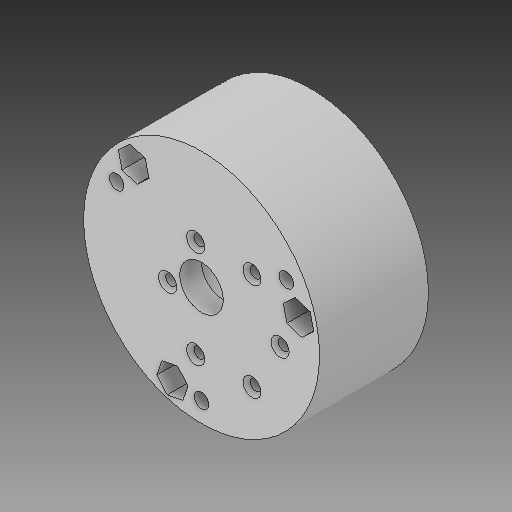
# Autodesk Inventor part: наболдашник
Saved by Autodesk Inventor 2019 (Build 230136000, 136)
## iProperties
Created: 2018-01-15
Part Number: наболдашник
Material: Типовые
Document SubType Name: Modeling
Designer: olege
Density: 1 g/cm^3
Appearance: По умолчанию
Mass: 53.9345 g
Surface Area: 284.424 cm^2
Volume: 53.9345 cm^3
Author: olege
Autodesk Inventor part; units mm, degrees
ref_plane "YZ Plane" through (0, 0, 0) normal (1, 0, 0) x (0, 1, 0)
ref_plane "XZ Plane" through (0, 0, 0) normal (0, 1, 0) x (-1, 0, 0)
ref_plane "XY Plane" through (0, 0, 0) normal (0, 0, 1) x (1, 0, 0)
sketch "Эскиз1" plane through (0, 0, 0) normal (0, 0, 1) x (1, 0, 0)
  circle A0 centre (0, 0) radius 18.65
  circle A1 centre (0, 0) radius 20.5
  dimension "d0" = 37.3
  dimension "d1" = 41
  constraints: 2 centre point, 2 coincident
  measures "d0" diameter of A0
  measures "d1" diameter of A1
extrude "Выдавливание1" add sketch "Эскиз1" against normal blind 24
sketch "Эскиз2" plane through (0, 0, 0) normal (0, 0, 1) x (1, 0, 0)
  circle A0 centre (0, 0) radius 20.5
  dimension "d4" = 41
  constraints: 1 centre point, 1 coincident
  measures "d4" diameter of A0
extrude "Выдавливание2" add sketch "Эскиз2" along normal blind 2
sketch "Эскиз3" plane through (0, 0, 2) normal (0, 0, 1) x (1, 0, 0)
  circle A0 centre (15.5, 0) radius 1.5
  point P0 (0, 0)
  dimension "d9" = 3
  dimension "d10" = 15.5
  constraints: 1 centre point, 1 horizontal alignment
  measures "d9" diameter of A0
  measures "d10" distance of point (0, 0) A0.centre
extrude "Выдавливание3" cut sketch "Эскиз3" against normal blind 2
pattern_circular "Круговой массив1" count 6 over 360 about axis through (0, 0, 0) along (0, 0, -1) of "Выдавливание3"
sketch "Эскиз4" plane through (0, 0, 2) normal (0, 0, 1) x (1, 0, 0)
  circle A0 centre (-6.1423, 3.3574) radius 6
  circle A1 centre (-7.75, 13.4234) radius 1.5 projected
  point P0 (0, 0)
  dimension "d17" = 12
  dimension "d19" = 7
  dimension "d20" = 10.066
  constraints: 1 centre point
  measures "d17" diameter of A0
  measures "d19" distance of point (0, 0) A0.centre
  measures "d20" vertical distance of A0.centre A1.centre
extrude "Выдавливание4" cut sketch "Эскиз4" against normal blind 2 contours A0
sketch "Эскиз5" plane through (0, 0, 2) normal (0, 0, 1) x (1, 0, 0)
  circle A0 centre (-6.1423, 3.3574) radius 6 construction
  circle A1 centre (-6.1423, 3.3574) radius 32.5
  circle A2 centre (0, 0) radius 20.5 projected
  dimension "d48" = 65
  constraints: 1 centre point, 1 coincident
  measures "d48" diameter of A1
extrude "Выдавливание5" add sketch "Эскиз5" against normal blind 2
sketch "Эскиз6" plane through (-6.1423, 3.3574, 0) normal (0, 0, -1) x (-1, 0, 0)
  circle A0 centre (0, 0) radius 32.5
  circle A1 centre (0, 0) radius 25.5
  point P0 (-6.1423, -3.3574)
  dimension "d25" = 51
  dimension "d26" = 65
  constraints: 2 centre point, 1 coincident
  measures "d25" diameter of A1
  measures "d26" diameter of A0
extrude "Выдавливание6" add sketch "Эскиз6" along normal blind 24
sketch "Эскиз8" plane through (0, 0, -24) normal (0, 0, -1) x (-1, 0, 0)
  circle A0 centre (0, 0) radius 18.65
  circle A1 centre (6.1423, 3.3574) radius 6 projected
  circle A2 centre (6.1423, 3.3574) radius 32.5
  circle A3 centre (6.1423, 3.3574) radius 35
  dimension "d33" = 65
  dimension "d34" = 70
  dimension "d209" = 37.3
  constraints: 3 centre point, 3 coincident
  measures "d33" diameter of A2
  measures "d34" diameter of A3
  measures "d209" diameter of A0
extrude "Выдавливание7" cut sketch "Эскиз8" against normal blind 25 contours A0 | A1 | A3
sketch "Эскиз10" plane through (0, 0, 1) normal (0, 0, -1) x (-1, 0, 0)
  circle A0 centre (6.1423, 3.3574) radius 6 projected
  circle A1 centre (-7.75, 13.4234) radius 1.5 projected
  circle A2 centre (7.75, 13.4234) radius 1.5 projected
  circle A3 centre (15.5, 0) radius 1.5 projected
  circle A4 centre (7.75, -13.4234) radius 1.5 projected
  circle A5 centre (-7.75, -13.4234) radius 1.5 projected
  circle A6 centre (-15.5, 0) radius 1.5 projected
  circle A7 centre (0, 0) radius 18.65 projected
extrude "Выдавливание9" add sketch "Эскиз10" along normal blind 1
sketch "Эскиз12" plane through (0, 0, 2) normal (0, 0, 1) x (1, 0, 0)
  circle A0 centre (-6.1423, 3.3574) radius 6 projected
  circle A1 centre (7.75, 13.4234) radius 1.5 projected
  circle A2 centre (-7.75, 13.4234) radius 1.5 projected
  circle A3 centre (-15.5, 0) radius 1.5 projected
  circle A4 centre (-7.75, -13.4234) radius 1.5 projected
  circle A5 centre (7.75, -13.4234) radius 1.5 projected
  circle A6 centre (15.5, 0) radius 1.5 projected
  circle A7 centre (-6.1423, 3.3574) radius 32.5 projected
  point P0 (0, 0)
extrude "Выдавливание10" add sketch "Эскиз12" along normal blind 4
chamfer "Фаска2" distance 1 angle 45 6 edges at (6.25, -13.4234, 6) (-9.25, -13.4234, 6) (-17, 0, 6) (-9.25, 13.4234, 6) (6.25, 13.4234, 6) (14, 0, 6)
sketch "Эскиз39" plane through (0, 0, 0) normal (0, 0, -1) x (-1, 0, 0)
  arc A0 (-3.714, -20.1608) -> (-18.9749, 7.759) centre (6.1423, 3.3574) ccw projected
  arc A1 (-3.714, -20.1608) -> (-18.9749, 7.759) centre (0, 0) ccw projected
extrude "Выдавливание31" add sketch "Эскиз39" along normal blind 24
sketch "Эскиз15" plane through (-6.1423, 3.3574, -24) normal (0, 0, -1) x (-1, 0, 0)
  line L0 (0, 0) -> (0, -9.4762) construction
  line L1 (0, 0) -> (-43.3013, 25) construction
  line L2 (0, 0) -> (50, 0) construction
  line L3 (-26.8827, 11.4793) -> (-26.8827, 15.5207)
  line L4 (-26.8827, 15.5207) -> (-23.3827, 17.5415)
  line L5 (-23.3827, 17.5415) -> (-19.8827, 15.5207)
  line L6 (-19.8827, 15.5207) -> (-19.8827, 11.4793)
  line L7 (-19.8827, 11.4793) -> (-23.3827, 9.4585)
  line L8 (-23.3827, 9.4585) -> (-26.8827, 11.4793)
  point P0 (-6.1423, -3.3574)
  point P1 (-23.3827, 13.5)
  dimension "d83" = 50
  dimension "d85" = 27
  dimension "d86" = 7
  dimension "d87" = 120
  constraints: 18 end point, 1 coincident, 1 equal length, 1 horizontal, 1 parallel, 1 point on line, 1 vertical, 14 other
  measures "d83" distance of L0.start L1.end
  measures "d85" distance of L0.start point (-23.383, 13.5)
  measures "d86" distance between parallel lines of L5 L8
  measures "d87" angle of L1 L0
extrude "Выдавливание13" cut sketch "Эскиз15" against normal blind 24
pattern_circular "Круговой массив3" count 3 over 360 about axis through (-6.1423, 3.3574, 2) along (0, 0, -1) of "Выдавливание13"
sketch "Эскиз16" plane through (-6.1423, 3.3574, 0) normal (0, 0, -1) x (-1, 0, 0)
  line L0 (-26.8827, 11.4793) -> (-26.8827, 15.5207) construction
  line L1 (-23.3827, 9.4585) -> (-26.8827, 11.4793) construction
  line L2 (-19.8827, 11.4793) -> (-23.3827, 9.4585) construction
  line L3 (-19.8827, 15.5207) -> (-19.8827, 11.4793) construction
  line L4 (-23.3827, 17.5415) -> (-19.8827, 15.5207) construction
  line L5 (-26.8827, 15.5207) -> (-23.3827, 17.5415) construction
  line L6 (-19.8827, 11.4793) -> (-23.3827, 9.4585) construction
  line L7 (-23.3827, 9.4585) -> (-26.8827, 11.4793) construction
  line L8 (-26.8827, 11.4793) -> (-26.8827, 15.5207) construction
  line L9 (-26.8827, 15.5207) -> (-23.3827, 17.5415) construction
  line L10 (-23.3827, 17.5415) -> (-19.8827, 15.5207) construction
  line L11 (-19.8827, 15.5207) -> (-19.8827, 11.4793) construction
  circle A0 centre (-23.3827, 13.5) radius 2
  point P0 (-6.1423, -3.3574)
  dimension "d94" = 4
  constraints: 12 end point, 1 centre point, 1 coincident, 13 other
  measures "d94" diameter of A0
extrude "Выдавливание14" cut sketch "Эскиз16" against normal blind 27
pattern_circular "Круговой массив4" count 3 over 360 about axis through (-6.1423, 3.3574, 2) along (0, 0, -1) of "Выдавливание14"
sketch "Эскиз28" plane through (-6.1423, 3.3574, 6) normal (0, 0, 1) x (1, 0, 0)
  line L0 (-17.7941, 16.1189) -> (-21.6589, 17.3005)
  line L1 (-21.6589, 17.3005) -> (-22.5681, 21.2384)
  line L2 (-22.5681, 21.2384) -> (-19.6123, 23.9946)
  line L3 (-19.6123, 23.9946) -> (-15.7475, 22.813)
  line L4 (-15.7475, 22.813) -> (-14.8384, 18.8751)
  line L5 (-14.8384, 18.8751) -> (-17.7941, 16.1189)
  line L6 (-18.7032, 20.0567) -> (26.7213, 6.1691) construction
  line L7 (26.7213, 6.1691) -> (-8.018, -26.2258) construction
  line L8 (-8.018, -26.2258) -> (-18.7032, 20.0567) construction
  line L9 (0, 0) -> (14.2356, 0) construction
  line L10 (-10.6581, -23.1658) -> (-6.688, -22.4095)
  line L11 (-6.688, -22.4095) -> (-4.048, -25.4695)
  line L12 (-4.048, -25.4695) -> (-5.378, -29.2858)
  line L13 (-5.378, -29.2858) -> (-9.3481, -30.0422)
  line L14 (-9.3481, -30.0422) -> (-11.9881, -26.9822)
  line L15 (-11.9881, -26.9822) -> (-10.6581, -23.1658)
  line L16 (25.8121, 10.107) -> (29.677, 8.9254)
  line L17 (29.677, 8.9254) -> (30.5861, 4.9875)
  line L18 (30.5861, 4.9875) -> (27.6304, 2.2312)
  line L19 (27.6304, 2.2312) -> (23.7655, 3.4128)
  line L20 (23.7655, 3.4128) -> (22.8564, 7.3507)
  line L21 (22.8564, 7.3507) -> (25.8121, 10.107)
  point P0 (6.1423, -3.3574)
  point P1 (-18.7032, 20.0567)
  point P2 (26.7213, 6.1691)
  dimension "d182" = 47.5
  dimension "d183" = 7
  dimension "d185" = 17
  dimension "d186" = 7
  dimension "d187" = 7
  constraints: 44 end point, 4 coincident, 1 collinear, 1 horizontal, 1 parallel, 47 other
  measures "d182" distance of L6.start L6.end
  measures "d183" distance between parallel lines of L5 L2
  measures "d185" angle of L6 L9
  measures "d186" distance between parallel lines of L12 L15
  measures "d187" distance between parallel lines of L19 L16
extrude "Выдавливание21" cut sketch "Эскиз28" against normal blind 31.25
sketch "Эскиз29" plane through (-6.1423, 3.3574, -24) normal (0, 0, -1) x (-1, 0, 0)
  circle A0 centre (-6.1423, -3.3574) radius 18.65 construction
  line L0 (10.6581, -23.1658) -> (11.9881, -26.9822) construction
  line L1 (11.9881, -26.9822) -> (9.3481, -30.0422) construction
  line L2 (9.3481, -30.0422) -> (5.378, -29.2858) construction
  line L3 (5.378, -29.2858) -> (4.048, -25.4695) construction
  line L4 (4.048, -25.4695) -> (6.688, -22.4095) construction
  line L5 (3.5, -24.9793) -> (3.5, -29.0207) construction
  line L6 (3.5, -29.0207) -> (0, -31.0415) construction
  line L7 (0, -31.0415) -> (-3.5, -29.0207) construction
  line L8 (-3.5, -29.0207) -> (-3.5, -24.9793) construction
  circle A1 centre (0, 0) radius 32.5 construction
  line L9 (-25.8121, 10.107) -> (-22.8564, 7.3507) construction
  line L10 (-23.3827, 9.4585) -> (-26.8827, 11.4793) construction
  line L11 (-26.8827, 11.4793) -> (-26.8827, 15.5207) construction
  line L12 (-26.8827, 15.5207) -> (-23.3827, 17.5415) construction
  line L13 (-23.3827, 17.5415) -> (-19.8827, 15.5207) construction
  line L14 (-19.8827, 15.5207) -> (-19.8827, 11.4793) construction
  line L15 (-19.8827, 11.4793) -> (-23.3827, 9.4585) construction
  line L16 (-22.8564, 7.3507) -> (-23.7655, 3.4128) construction
  line L17 (-23.7655, 3.4128) -> (-27.6304, 2.2312) construction
  line L18 (-27.6304, 2.2312) -> (-30.5861, 4.9875) construction
  line L19 (-30.5861, 4.9875) -> (-29.677, 8.9254) construction
  line L20 (-29.677, 8.9254) -> (-25.8121, 10.107) construction
  line L21 (14.8384, 18.8751) -> (15.7475, 22.813) construction
  line L22 (15.7475, 22.813) -> (19.6123, 23.9946) construction
  line L23 (19.6123, 23.9946) -> (22.5681, 21.2384) construction
  line L24 (22.5681, 21.2384) -> (21.6589, 17.3005) construction
  line L25 (21.6589, 17.3005) -> (17.7941, 16.1189) construction
  line L26 (19.8827, 15.5207) -> (23.3827, 17.5415) construction
  line L27 (23.3827, 17.5415) -> (26.8827, 15.5207) construction
  line L28 (26.8827, 15.5207) -> (26.8827, 11.4793) construction
  line L29 (26.8827, 11.4793) -> (23.3827, 9.4585) construction
  line L30 (10.6581, -23.1658) -> (5.378, -29.2858) construction
  line L31 (8.018, -26.2258) -> (-26.7213, 6.1691) construction
  line L32 (-26.7213, 6.1691) -> (18.7032, 20.0567) construction
  line L33 (18.7032, 20.0567) -> (8.018, -26.2258) construction
  line L34 (5.378, -29.2858) -> (4.048, -25.4695) projected
  line L35 (5.378, -29.2858) -> (4.048, -25.4695)
  line L36 (4.048, -25.4695) -> (6.688, -22.4095)
  line L37 (6.688, -22.4095) -> (10.6581, -23.1658)
  line L38 (10.6581, -23.1658) -> (11.9881, -26.9822)
  line L39 (11.9881, -26.9822) -> (9.3481, -30.0422)
  line L40 (9.3481, -30.0422) -> (5.378, -29.2858)
  line L41 (-27.6304, 2.2312) -> (-23.7655, 3.4128)
  line L42 (-27.6304, 2.2312) -> (-30.5861, 4.9875)
  line L43 (-30.5861, 4.9875) -> (-29.677, 8.9254)
  line L44 (-29.677, 8.9254) -> (-25.8121, 10.107)
  line L45 (-25.8121, 10.107) -> (-22.8564, 7.3507)
  line L46 (-22.8564, 7.3507) -> (-23.7655, 3.4128)
  line L47 (-23.7655, 3.4128) -> (-27.6304, 2.2312)
  line L48 (14.8384, 18.8751) -> (15.7475, 22.813) projected
  line L49 (15.7475, 22.813) -> (19.6123, 23.9946)
  line L50 (19.6123, 23.9946) -> (22.5681, 21.2384)
  line L51 (22.5681, 21.2384) -> (21.6589, 17.3005)
  line L52 (21.6589, 17.3005) -> (17.7941, 16.1189)
  line L53 (17.7941, 16.1189) -> (14.8384, 18.8751)
  line L54 (14.8384, 18.8751) -> (15.7475, 22.813)
  line L55 (23.6723, 21.576) -> (19.8721, 25.1197)
  line L56 (19.8721, 25.1197) -> (14.903, 23.6005)
  line L57 (14.903, 23.6005) -> (13.7341, 18.5375)
  line L58 (13.7341, 18.5375) -> (17.5343, 14.9938)
  line L59 (17.5343, 14.9938) -> (22.5034, 16.513)
  line L60 (22.5034, 16.513) -> (23.6723, 21.576)
  line L61 (6.365, -21.4827) -> (3.0838, -25.2858)
  line L62 (3.0838, -25.2858) -> (4.7369, -30.029)
  line L63 (4.7369, -30.029) -> (9.6711, -30.969)
  line L64 (9.6711, -30.969) -> (12.9522, -27.1658)
  line L65 (12.9522, -27.1658) -> (11.2992, -22.4227)
  line L66 (11.2992, -22.4227) -> (6.365, -21.4827)
  line L67 (-23.6246, 9.5982) -> (-26.8827, 11.4793) projected
  line L68 (-26.7213, 11.3861) -> (-22.2032, 8.7776)
  line L69 (-22.2032, 8.7776) -> (-22.2032, 3.5606)
  line L70 (-22.2032, 3.5606) -> (-26.7213, 0.9521)
  line L71 (-26.7213, 0.9521) -> (-31.2393, 3.5606)
  line L72 (-31.2393, 3.5606) -> (-31.2393, 8.7776)
  line L73 (-31.2393, 8.7776) -> (-26.7213, 11.3861)
  line L74 (6.688, -22.4095) -> (10.6581, -23.1658) projected
  line L75 (17.7941, 16.1189) -> (14.8384, 18.8751) projected
  line L76 (23.3827, 9.4585) -> (19.8827, 11.4793) projected
  line L77 (19.8827, 11.4793) -> (19.8827, 15.5207) projected
  line L78 (-3.5, -24.9793) -> (0, -22.9585) projected
  line L79 (0, -22.9585) -> (3.5, -24.9793) projected
  point P0 (15.2065, 20.4698)
  dimension "d190" = 1
  dimension "d191" = 0.85
  constraints: 82 end point, 4 coincident, 1 midpoint, 1 point on line, 69 other
  measures "d190" distance between parallel lines of L50 L55
  measures "d191" distance between parallel lines of L36 L61
extrude "Выдавливание22" add sketch "Эскиз29" against normal blind 30
sketch "Эскиз30" plane through (0, 0, 0) normal (0, 0, -1) x (-1, 0, 0)
  circle A0 centre (0, 0) radius 18.65
  dimension "d195" = 37.3
  constraints: 1 centre point, 1 coincident
  measures "d195" diameter of A0
extrude "Выдавливание23" cut sketch "Эскиз30" along normal blind 30
sketch "Эскиз31" plane through (-6.1423, 3.3574, -24) normal (0, 0, -1) x (-1, 0, 0)
  line L0 (-29.677, 8.9254) -> (-25.8121, 10.107) projected
  line L1 (-30.5861, 4.9875) -> (-29.677, 8.9254) projected
  line L2 (-27.6304, 2.2312) -> (-30.5861, 4.9875) projected
  line L3 (-23.7655, 3.4128) -> (-27.6304, 2.2312) projected
  line L4 (-22.8564, 7.3507) -> (-23.7655, 3.4128) projected
  line L5 (-25.8121, 10.107) -> (-22.8564, 7.3507) projected
  line L6 (17.7941, 16.1189) -> (14.8384, 18.8751) projected
  line L7 (21.6589, 17.3005) -> (17.7941, 16.1189) projected
  line L8 (22.5681, 21.2384) -> (21.6589, 17.3005) projected
  line L9 (19.6123, 23.9946) -> (22.5681, 21.2384) projected
  line L10 (15.7475, 22.813) -> (19.6123, 23.9946) projected
  line L11 (14.8384, 18.8751) -> (15.7475, 22.813) projected
  line L12 (4.048, -25.4695) -> (6.688, -22.4095) projected
  line L13 (6.688, -22.4095) -> (10.6581, -23.1658) projected
  line L14 (10.6581, -23.1658) -> (11.9881, -26.9822) projected
  line L15 (11.9881, -26.9822) -> (9.3481, -30.0422) projected
  line L16 (9.3481, -30.0422) -> (5.378, -29.2858) projected
  line L17 (5.378, -29.2858) -> (4.048, -25.4695) projected
  circle A0 centre (8.018, -26.2258) radius 2
  line L18 (14.8384, 18.8751) -> (22.5681, 21.2384) construction
  line L19 (21.6589, 17.3005) -> (15.7475, 22.813) construction
  line L20 (19.6123, 23.9946) -> (15.7475, 22.813) projected
  line L21 (19.6123, 23.9946) -> (17.7941, 16.1189) construction
  circle A1 centre (18.7032, 20.0567) radius 2
  line L22 (4.048, -25.4695) -> (11.9881, -26.9822) construction
  line L23 (10.6581, -23.1658) -> (5.378, -29.2858) construction
  line L24 (9.3481, -30.0422) -> (6.688, -22.4095) construction
  line L25 (-23.7655, 3.4128) -> (-22.8564, 7.3507) construction
  line L26 (-30.5861, 4.9875) -> (-22.8564, 7.3507) construction
  line L27 (-27.6304, 2.2312) -> (-25.8121, 10.107) construction
  line L28 (-29.677, 8.9254) -> (-23.7655, 3.4128) construction
  circle A2 centre (-26.7213, 6.1691) radius 2
  point P0 (-6.1423, -3.3574)
  dimension "d198" = 4
  dimension "d199" = 4
  dimension "d200" = 4
  constraints: 18 end point, 3 centre point, 3 midpoint, 1 coincident
  measures "d198" diameter of A0
  measures "d199" diameter of A1
  measures "d200" diameter of A2
extrude "Выдавливание24" add sketch "Эскиз31" against normal blind 6
sketch "Эскиз32" plane through (-26.025, 14.8367, 0) normal (0, 0, -1) x (-1, 0, 0)
  circle A0 centre (3.5, 2.0207) radius 2 construction
  line L0 (7, 4.0415) -> (7, 0) projected
  line L1 (7, 0) -> (3.5, -2.0207)
  line L2 (3.5, -2.0207) -> (0, 0)
  line L3 (0, 0) -> (0, 4.0415)
  line L4 (0, 4.0415) -> (3.5, 6.0622)
  line L5 (3.5, 6.0622) -> (7, 4.0415)
  line L6 (7, 4.0415) -> (7, 0)
  circle A1 centre (-19.8827, -38.4793) radius 2 construction
  line L7 (-19.8827, -42.5207) -> (-23.3827, -40.5)
  line L8 (-23.3827, -40.5) -> (-23.3827, -36.4585)
  line L9 (-23.3827, -36.4585) -> (-19.8827, -34.4378)
  line L10 (-19.8827, -34.4378) -> (-16.3827, -36.4585)
  line L11 (-16.3827, -36.4585) -> (-16.3827, -40.5)
  line L12 (-16.3827, -40.5) -> (-19.8827, -42.5207)
  point P0 (-26.025, -14.8367)
  constraints: 24 end point, 2 coincident, 26 other
extrude "Выдавливание25" cut sketch "Эскиз32" along normal blind 139
sketch "Эскиз35" plane through (-6.1423, 3.3574, 6) normal (0, 0, 1) x (1, 0, 0)
  circle A0 centre (-8.018, -26.2258) radius 2 projected
  circle A1 centre (-8.018, -26.2258) radius 4.75
  point P0 (6.1423, -3.3574)
  dimension "d210" = 9.5
  constraints: 1 centre point, 1 coincident
  measures "d210" diameter of A1
sketch "Эскиз36" plane through (-6.1423, 3.3574, 6) normal (0, 0, 1) x (1, 0, 0)
  circle A0 centre (-8.018, -26.2258) radius 2 projected
  line L0 (-9.3481, -30.0422) -> (-11.9881, -26.9822) projected
  line L1 (-9.3481, -30.0422) -> (-11.9881, -26.9822)
  line L2 (-11.9881, -26.9822) -> (-10.6581, -23.1658)
  line L3 (-10.6581, -23.1658) -> (-6.688, -22.4095)
  line L4 (-6.688, -22.4095) -> (-4.048, -25.4695)
  line L5 (-4.048, -25.4695) -> (-5.378, -29.2858)
  line L6 (-5.378, -29.2858) -> (-9.3481, -30.0422)
  line L7 (-10.8844, -22.9035) -> (-12.3284, -27.047)
  line L8 (-12.3284, -27.047) -> (-9.4621, -30.3693)
  line L9 (-9.4621, -30.3693) -> (-5.1517, -29.5481)
  line L10 (-5.1517, -29.5481) -> (-3.7077, -25.4047)
  line L11 (-3.7077, -25.4047) -> (-6.574, -22.0824)
  line L12 (-6.574, -22.0824) -> (-10.8844, -22.9035)
  point P0 (6.1423, -3.3574)
  dimension "d212" = 0.3
  constraints: 24 end point, 2 coincident, 18 other
  measures "d212" distance between parallel lines of L2 L7
extrude "Выдавливание28" cut sketch "Эскиз36" against normal blind 24 contours L0 L2 L3 L4 L5 L6 | L12 L11 L10 L9 L8 L7
sketch "Эскиз37" plane through (-6.1423, 3.3574, 6) normal (0, 0, 1) x (1, 0, 0)
  circle A0 centre (26.7213, 6.1691) radius 2 projected
  circle A1 centre (-18.7032, 20.0567) radius 2 projected
  circle A2 centre (26.7213, 6.1691) radius 2 projected
  line L0 (25.8121, 10.107) -> (29.677, 8.9254) projected
  line L1 (22.8564, 7.3507) -> (25.8121, 10.107) projected
  line L2 (23.7655, 3.4128) -> (22.8564, 7.3507) projected
  line L3 (27.6304, 2.2312) -> (23.7655, 3.4128) projected
  line L4 (30.5861, 4.9875) -> (27.6304, 2.2312) projected
  line L5 (29.677, 8.9254) -> (30.5861, 4.9875) projected
  line L6 (27.7083, 1.8937) -> (23.5122, 3.1766)
  line L7 (23.5122, 3.1766) -> (22.5251, 7.452)
  line L8 (22.5251, 7.452) -> (25.7342, 10.4445)
  line L9 (25.7342, 10.4445) -> (29.9303, 9.1616)
  line L10 (29.9303, 9.1616) -> (30.9174, 4.8862)
  line L11 (30.9174, 4.8862) -> (27.7083, 1.8937)
  line L12 (-17.7941, 16.1189) -> (-21.6589, 17.3005) projected
  line L13 (-14.8384, 18.8751) -> (-17.7941, 16.1189) projected
  line L14 (-15.7475, 22.813) -> (-14.8384, 18.8751) projected
  line L15 (-19.6123, 23.9946) -> (-15.7475, 22.813) projected
  line L16 (-22.5681, 21.2384) -> (-19.6123, 23.9946) projected
  line L17 (-21.6589, 17.3005) -> (-22.5681, 21.2384) projected
  circle A3 centre (-18.7032, 20.0567) radius 2 projected
  line L18 (-17.7162, 15.7813) -> (-21.9123, 17.0642)
  line L19 (-21.9123, 17.0642) -> (-22.8994, 21.3396)
  line L20 (-22.8994, 21.3396) -> (-19.6903, 24.3321)
  line L21 (-19.6903, 24.3321) -> (-15.4941, 23.0493)
  line L22 (-15.4941, 23.0493) -> (-14.5071, 18.7739)
  line L23 (-14.5071, 18.7739) -> (-17.7162, 15.7813)
  point P0 (6.1423, -3.3574)
  dimension "d215" = 0.3
  dimension "d216" = 0.3
  constraints: 24 end point, 10 other
  measures "d215" distance between parallel lines of L4 L11
  measures "d216" distance between parallel lines of L13 L23
extrude "Выдавливание29" cut sketch "Эскиз37" against normal blind 24 contours L6 L7 L8 L9 L10 L11 | L18 L19 L20 L21 L22 L23
sketch "Эскиз38" plane through (-6.1423, 3.3574, -24) normal (0, 0, -1) x (-1, 0, 0)
  circle A0 centre (-23.3827, 13.5) radius 2 projected
  line L0 (-26.8827, 11.4793) -> (-26.8827, 15.5207)
  line L1 (-26.8827, 15.5207) -> (-23.3827, 17.5415)
  line L2 (-23.3827, 17.5415) -> (-19.8827, 15.5207)
  line L3 (-19.8827, 15.5207) -> (-19.8827, 11.4793)
  line L4 (-19.8827, 11.4793) -> (-23.3827, 9.4585)
  line L5 (-23.3827, 9.4585) -> (-26.8827, 11.4793)
  line L6 (23.3827, 17.5415) -> (19.8827, 15.5207) projected
  line L7 (19.8827, 15.5207) -> (19.8827, 11.4793) projected
  line L8 (19.8827, 11.4793) -> (23.3827, 9.4585) projected
  line L9 (26.8827, 11.4793) -> (23.3827, 9.4585) projected
  line L10 (26.8827, 15.5207) -> (26.8827, 11.4793) projected
  line L11 (23.3827, 17.5415) -> (26.8827, 15.5207) projected
  circle A1 centre (23.3827, 13.5) radius 2 projected
  circle A2 centre (0, -27) radius 2 projected
  line L12 (-3.5, -29.0207) -> (-3.5, -24.9793) projected
  line L13 (-3.5, -29.0207) -> (-3.5, -24.9793)
  line L14 (-3.5, -24.9793) -> (0, -22.9585)
  line L15 (0, -22.9585) -> (3.5, -24.9793)
  line L16 (3.5, -24.9793) -> (3.5, -29.0207)
  line L17 (3.5, -29.0207) -> (0, -31.0415)
  line L18 (0, -31.0415) -> (-3.5, -29.0207)
  line L19 (-3.8, -29.1939) -> (-3.8, -24.8061)
  line L20 (-3.8, -24.8061) -> (0, -22.6121)
  line L21 (0, -22.6121) -> (3.8, -24.8061)
  line L22 (3.8, -24.8061) -> (3.8, -29.1939)
  line L23 (3.8, -29.1939) -> (0, -31.3879)
  line L24 (0, -31.3879) -> (-3.8, -29.1939)
  line L25 (19.5827, 15.6939) -> (23.3827, 17.8879)
  line L26 (23.3827, 17.8879) -> (27.1827, 15.6939)
  line L27 (27.1827, 15.6939) -> (27.1827, 11.3061)
  line L28 (27.1827, 11.3061) -> (23.3827, 9.1121)
  line L29 (23.3827, 9.1121) -> (19.5827, 11.3061)
  line L30 (19.5827, 11.3061) -> (19.5827, 15.6939)
  line L31 (-19.5827, 15.6939) -> (-23.3827, 17.8879)
  line L32 (-23.3827, 17.8879) -> (-27.1827, 15.6939)
  line L33 (-27.1827, 15.6939) -> (-27.1827, 11.3061)
  line L34 (-27.1827, 11.3061) -> (-23.3827, 9.1121)
  line L35 (-23.3827, 9.1121) -> (-19.5827, 11.3061)
  line L36 (-19.5827, 11.3061) -> (-19.5827, 15.6939)
  point P0 (-6.1423, -3.3574)
  point P1 (-3.5, -25.2587)
  dimension "d219" = 0.3
  dimension "d220" = 0.3
  dimension "d221" = 0.3
  constraints: 60 end point, 2 coincident, 41 other
  measures "d219" distance between parallel lines of L18 L24
  measures "d220" distance between parallel lines of L6 L25
  measures "d221" distance between parallel lines of L2 L31
extrude "Выдавливание30" cut sketch "Эскиз38" against normal blind 24 contours L19 L20 L21 L22 L23 L24 | L25 L26 L27 L28 L29 L30 | L36 L35 L34 L33 L32 L31
